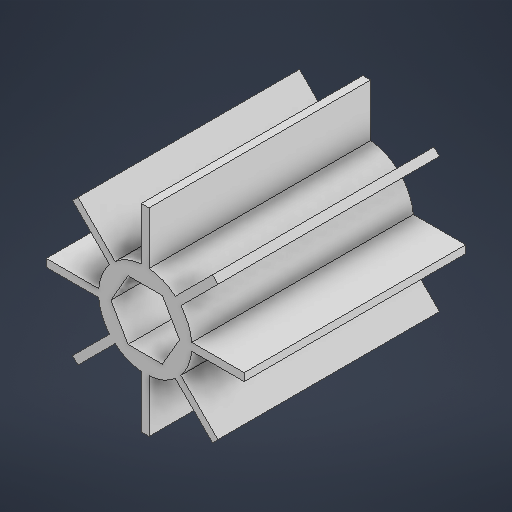
# Autodesk Inventor part: Spiral
Saved by Autodesk Inventor 2026 (Build 300175050, 175E)
## iProperties
Created: 2025-11-03
Part Number: Spiral
Material: Generic
Document SubType Name: Modeling
Designer: randy
Density: 1 g/cm^3
Appearance: Default
Author: randy
Autodesk Inventor part; units mm, degrees
ref_plane "YZ Plane" through (0, 0, 0) normal (1, 0, 0) x (0, 1, 0)
ref_plane "XZ Plane" through (0, 0, 0) normal (0, 1, 0) x (-1, 0, 0)
ref_plane "XY Plane" through (0, 0, 0) normal (0, 0, 1) x (1, 0, 0)
sketch "Sketch1" plane through (0, 0, 0) normal (0, 0, 1) x (1, 0, 0)
  circle A0 centre (0, 0) radius 10.16
  circle A1 centre (0, 0) radius 8.5725
  line L0 (0.8382, 10.1254) -> (0.8382, 21.5554)
  line L1 (0.8382, 21.5554) -> (-0.8382, 21.5554)
  line L2 (-0.8382, 21.5554) -> (-0.8382, 10.1254)
  line L3 (-15.8346, 14.6492) -> (-7.7524, 6.567)
  line L4 (-14.6492, 15.8346) -> (-15.8346, 14.6492)
  line L5 (-6.567, 7.7524) -> (-14.6492, 15.8346)
  line L6 (-21.5554, -0.8382) -> (-10.1254, -0.8382)
  line L7 (-21.5554, 0.8382) -> (-21.5554, -0.8382)
  line L8 (-10.1254, 0.8382) -> (-21.5554, 0.8382)
  line L9 (-14.6492, -15.8346) -> (-6.567, -7.7524)
  line L10 (-15.8346, -14.6492) -> (-14.6492, -15.8346)
  line L11 (-7.7524, -6.567) -> (-15.8346, -14.6492)
  line L12 (0.8382, -21.5554) -> (0.8382, -10.1254)
  line L13 (-0.8382, -21.5554) -> (0.8382, -21.5554)
  line L14 (-0.8382, -10.1254) -> (-0.8382, -21.5554)
  line L15 (15.8346, -14.6492) -> (7.7524, -6.567)
  line L16 (14.6492, -15.8346) -> (15.8346, -14.6492)
  line L17 (6.567, -7.7524) -> (14.6492, -15.8346)
  line L18 (21.5554, 0.8382) -> (10.1254, 0.8382)
  line L19 (21.5554, -0.8382) -> (21.5554, 0.8382)
  line L20 (10.1254, -0.8382) -> (21.5554, -0.8382)
  line L21 (14.6492, 15.8346) -> (6.567, 7.7524)
  line L22 (15.8346, 14.6492) -> (14.6492, 15.8346)
  line L23 (7.7524, 6.567) -> (15.8346, 14.6492)
  line L24 (-7.479, 0) -> (-3.7395, 6.477)
  line L25 (-3.7395, 6.477) -> (3.7395, 6.477)
  line L26 (3.7395, 6.477) -> (7.479, 0)
  line L27 (7.479, 0) -> (3.7395, -6.477)
  line L28 (3.7395, -6.477) -> (-3.7395, -6.477)
  line L29 (-3.7395, -6.477) -> (-7.479, 0)
  point P0 (0, 21.5554)
  point P1 (-15.2419, 15.2419)
  point P2 (-21.5554, 0)
  point P3 (-15.2419, -15.2419)
  point P4 (0, -21.5554)
  point P5 (15.2419, -15.2419)
  point P6 (21.5554, 0)
  point P7 (15.2419, 15.2419)
  point P8 (-10.1254, -0.8382)
  point P9 (-10.1254, 0.8382)
  point P10 (-6.567, -7.7524)
  point P11 (-7.7524, -6.567)
  point P12 (0.8382, -10.1254)
  point P13 (-0.8382, -10.1254)
  point P14 (7.7524, -6.567)
  point P15 (6.567, -7.7524)
  point P16 (10.1254, 0.8382)
  point P17 (10.1254, -0.8382)
  point P18 (6.567, 7.7524)
  point P19 (7.7524, 6.567)
  point P20 (-7.7524, 6.567)
  point P21 (-6.567, 7.7524)
  dimension "d0" = 20.32
  dimension "d1" = 1.5875
  dimension "d7" = 1.6764
  dimension "d11" = 360
  dimension "d13" = 11.43
  dimension "d17" = 12.954
  constraints: 60 end point, 2 centre point, 2 coincident, 2 parallel, 2 point on circle, 1 horizontal, 1 midpoint, 1 perpendicular, 1 vertical alignment, 78 other
  measures "d0" diameter of A0
  measures "d1" radial gap between concentric circles of A0 A1
  measures "d7" distance between parallel lines of L2 L0
  measures "d13" distance of L0.start L0.end
  measures "d17" distance between parallel lines of L28 L25
extrude "Extrusion1" add sketch "Sketch1" along normal mid plane 48.26 contours A0 | A0 L18 L19 L20 | A0 L21 L22 L23 | L15 L16 L17 A0 | A0 L2 L1 L0 | L12 L13 L14 A0 | A0 L3 L4 L5 | L9 L10 L11 A0 | A0 L6 L7 L8 | A1
body "Solid1"
